Autodesk Inventor part; units mm, degrees
(part 2 of 2)
sketch "스케치7" plane through (-13.4999, 0, 82.7525) normal (-1, 0, 0) x (0, 0, -1)
  line L0 (22.7351, -5) -> (22.028, -5) projected
  line L1 (22.028, -5) -> (21.3209, -5) projected
  line L2 (21.3209, -5) -> (22.028, -5) projected
  line L3 (22.028, -5) -> (21.3209, -5) projected
  line L4 (21.3209, -5) -> (20.6138, -5) projected
  line L5 (20.6138, -5) -> (19.9067, -5) projected
  line L6 (19.9067, -5) -> (20.6138, -5) projected
  line L7 (20.6138, -5) -> (19.9067, -5) projected
  line L8 (19.9067, -5) -> (19.1996, -5) projected
  line L9 (19.1996, -5) -> (18.4924, -5) projected
  line L10 (18.4924, -5) -> (19.4924, -5) projected
  line L11 (19.4924, -5) -> (18.4924, -5) projected
  line L12 (18.4924, -5) -> (19.4924, -5) projected
  line L13 (19.4924, -5) -> (18.4924, -5) projected
  line L14 (18.4924, -5) -> (19.4924, -5) projected
  line L15 (19.4924, -5) -> (18.4924, -5) projected
  line L16 (18.4924, -5) -> (19.4924, -5) projected
  line L17 (19.4924, -5) -> (18.4924, -5) projected
  line L18 (18.4924, -5) -> (19.4924, -5) projected
  line L19 (19.4924, -5) -> (18.4924, -5) projected
  line L20 (18.4924, -5) -> (19.4924, -5) projected
  line L21 (19.4924, -5) -> (18.4924, -5) projected
  line L22 (18.4924, -5) -> (19.4924, -5) projected
  line L23 (19.4924, -5) -> (18.4924, -5) projected
  line L24 (18.4924, -5) -> (19.4924, -5) projected
  line L25 (19.4924, -5) -> (18.4924, -5) projected
  line L26 (18.4924, -5) -> (19.4924, -5) projected
  line L27 (19.4924, -5) -> (18.4924, -5) projected
  line L28 (18.4924, -5) -> (19.4924, -5) projected
  line L29 (19.4924, -5) -> (18.4924, -5) projected
  line L30 (18.4924, -5) -> (19.4924, -5) projected
  line L31 (19.4924, -5) -> (18.4924, -5) projected
  line L32 (18.4924, -5) -> (19.4924, -5) projected
  line L33 (19.4924, -5) -> (18.4924, -5) projected
  line L34 (18.4924, -5) -> (20.0726, -5) projected
  line L35 (20.0726, -5) -> (20.7798, -5) projected
  line L36 (20.7798, -5) -> (21.4869, -5) projected
  line L37 (21.4869, -5) -> (20.7798, -5) projected
  line L38 (20.7798, -5) -> (21.4869, -5) projected
  line L39 (21.4869, -5) -> (22.194, -5) projected
  line L40 (22.194, -5) -> (22.9011, -5) projected
  line L41 (22.9011, -5) -> (22.194, -5) projected
  line L42 (22.194, -5) -> (22.9011, -5) projected
  line L43 (22.9011, -5) -> (23.6082, -5) projected
  line L44 (23.6082, -5) -> (24.3153, -5) projected
  line L45 (24.3153, -5) -> (23.6082, -5) projected
  line L46 (23.6082, -5) -> (24.3153, -5) projected
  line L47 (24.3153, -5) -> (25.0224, -5) projected
  line L48 (25.0224, -5) -> (25.7295, -5) projected
  line L49 (25.7295, -5) -> (25.0224, -5) projected
  line L50 (25.0224, -5) -> (25.7295, -5) projected
  line L51 (25.7295, -5) -> (26.4366, -5) projected
  line L52 (26.4366, -5) -> (27.1437, -5) projected
  line L53 (27.1437, -5) -> (26.4366, -5) projected
  line L54 (26.4366, -5) -> (27.1437, -5) projected
  line L55 (27.1437, -5) -> (27.8508, -5) projected
  line L56 (27.8508, -5) -> (28.5579, -5) projected
  line L57 (28.5579, -5) -> (27.8508, -5) projected
  line L58 (27.8508, -5) -> (28.5579, -5) projected
  line L59 (28.5579, -5) -> (29.265, -5) projected
  line L60 (29.265, -5) -> (29.9721, -5) projected
  line L61 (29.9721, -5) -> (29.265, -5) projected
  line L62 (29.265, -5) -> (29.9721, -5) projected
  line L63 (29.9721, -5) -> (30.6792, -5) projected
  line L64 (30.6792, -5) -> (31.3864, -5) projected
  line L65 (31.3864, -5) -> (30.6792, -5) projected
  line L66 (30.6792, -5) -> (31.3864, -5) projected
  line L67 (31.3864, -5) -> (32.0935, -5) projected
  line L68 (32.0935, -5) -> (32.8006, -5) projected
  line L69 (32.8006, -5) -> (32.0935, -5) projected
  line L70 (32.0935, -5) -> (32.8006, -5) projected
  line L71 (32.8006, -5) -> (33.5077, -5) projected
  line L72 (33.5077, -5) -> (34.2148, -5) projected
  line L73 (34.2148, -5) -> (33.5077, -5) projected
  line L74 (33.5077, -5) -> (34.2148, -5) projected
  line L75 (34.2148, -5) -> (34.9219, -5) projected
  line L76 (34.9219, -5) -> (35.629, -5) projected
  line L77 (35.629, -5) -> (34.9219, -5) projected
  line L78 (34.9219, -5) -> (35.629, -5) projected
  line L79 (35.629, -5) -> (36.3361, -5) projected
  line L80 (36.3361, -5) -> (37.0432, -5) projected
  line L81 (37.0432, -5) -> (36.3361, -5) projected
  line L82 (36.3361, -5) -> (37.0432, -5) projected
  line L83 (37.0432, -5) -> (39.2779, -5) projected
  line L84 (39.2779, -5) -> (40.2779, -5) projected
  line L85 (40.2779, -5) -> (41.2779, -5) projected
  line L86 (41.2779, -5) -> (42.2779, -5) projected
  line L87 (42.2779, -5) -> (43.2779, -5) projected
  line L88 (43.2779, -5) -> (44.2779, -5) projected
  line L89 (44.2779, -5) -> (45.2779, -5) projected
  line L90 (45.2779, -5) -> (46.2779, -5) projected
  line L91 (46.2779, -5) -> (47.2779, -5) projected
  line L92 (47.2779, -5) -> (48.2779, -5) projected
  line L93 (48.2779, -5) -> (49.2779, -5) projected
  line L94 (49.2779, -5) -> (50.2779, -5) projected
  line L95 (50.2779, -5) -> (51.2779, -5) projected
  line L96 (51.2779, -5) -> (52.2779, -5) projected
  line L97 (52.2779, -5) -> (53.2779, -5) projected
  line L98 (53.2779, -5) -> (54.2779, -5) projected
  line L99 (54.2779, -5) -> (55.2779, -5) projected
  line L100 (55.2779, -5) -> (56.2779, -5) projected
  line L101 (56.2779, -5) -> (57.2779, -5) projected
  line L102 (57.2779, -5) -> (58.2779, -5) projected
  line L103 (58.2779, -5) -> (59.2779, -5) projected
  line L104 (59.2779, -5) -> (60.2779, -5) projected
  line L105 (60.2779, -5) -> (61.2779, -5) projected
  line L106 (61.2779, -5) -> (62.2779, -5) projected
  line L107 (62.2779, -5) -> (63.2779, -5) projected
  line L108 (63.2779, -5) -> (64.8581, -5) projected
  line L109 (64.8581, -5) -> (64.151, -5) projected
  line L110 (64.151, -5) -> (64.8581, -5) projected
  line L111 (64.8581, -5) -> (65.5652, -5) projected
  line L112 (65.5652, -5) -> (66.2723, -5) projected
  line L113 (66.2723, -5) -> (65.5652, -5) projected
  line L114 (65.5652, -5) -> (66.2723, -5) projected
  line L115 (66.2723, -5) -> (66.9795, -5) projected
  line L116 (66.9795, -5) -> (67.6866, -5) projected
  line L117 (67.6866, -5) -> (66.9795, -5) projected
  line L118 (66.9795, -5) -> (67.6866, -5) projected
  line L119 (67.6866, -5) -> (68.3937, -5) projected
  line L120 (68.3937, -5) -> (69.1008, -5) projected
  line L121 (69.1008, -5) -> (68.3937, -5) projected
  line L122 (68.3937, -5) -> (69.1008, -5) projected
  line L123 (69.1008, -5) -> (69.8079, -5) projected
  line L124 (69.8079, -5) -> (70.515, -5) projected
  line L125 (70.515, -5) -> (69.8079, -5) projected
  line L126 (69.8079, -5) -> (70.515, -5) projected
  line L127 (70.515, -5) -> (71.2221, -5) projected
  line L128 (71.2221, -5) -> (71.9292, -5) projected
  line L129 (71.9292, -5) -> (71.2221, -5) projected
  line L130 (71.2221, -5) -> (71.9292, -5) projected
  line L131 (71.9292, -5) -> (72.6363, -5) projected
  line L132 (72.6363, -5) -> (73.3434, -5) projected
  line L133 (73.3434, -5) -> (72.6363, -5) projected
  line L134 (72.6363, -5) -> (73.3434, -5) projected
  line L135 (73.3434, -5) -> (74.0505, -5) projected
  line L136 (74.0505, -5) -> (74.7576, -5) projected
  line L137 (74.7576, -5) -> (74.0505, -5) projected
  line L138 (74.0505, -5) -> (74.7576, -5) projected
  line L139 (74.7576, -5) -> (75.4647, -5) projected
  line L140 (75.4647, -5) -> (76.1718, -5) projected
  line L141 (76.1718, -5) -> (75.4647, -5) projected
  line L142 (75.4647, -5) -> (76.1718, -5) projected
  line L143 (76.1718, -5) -> (76.8789, -5) projected
  line L144 (76.8789, -5) -> (77.5861, -5) projected
  line L145 (77.5861, -5) -> (76.8789, -5) projected
  line L146 (76.8789, -5) -> (77.5861, -5) projected
  line L147 (77.5861, -5) -> (78.2932, -5) projected
  line L148 (78.2932, -5) -> (79.0003, -5) projected
  line L149 (79.0003, -5) -> (78.2932, -5) projected
  line L150 (78.2932, -5) -> (79.0003, -5) projected
  line L151 (79.0003, -5) -> (79.7074, -5) projected
  line L152 (79.7074, -5) -> (80.4145, -5) projected
  line L153 (80.4145, -5) -> (79.7074, -5) projected
  line L154 (79.7074, -5) -> (80.4145, -5) projected
  line L155 (80.4145, -5) -> (81.1216, -5) projected
  line L156 (81.1216, -5) -> (81.8287, -5) projected
  line L157 (81.8287, -5) -> (80.8287, -5) projected
  line L158 (80.8287, -5) -> (81.8287, -5) projected
  line L159 (81.8287, -5) -> (80.8287, -5) projected
  line L160 (80.8287, -5) -> (81.8287, -5) projected
  line L161 (81.8287, -5) -> (80.8287, -5) projected
  line L162 (80.8287, -5) -> (81.8287, -5) projected
  line L163 (81.8287, -5) -> (80.8287, -5) projected
  line L164 (80.8287, -5) -> (81.8287, -5) projected
  line L165 (81.8287, -5) -> (80.8287, -5) projected
  line L166 (80.8287, -5) -> (81.8287, -5) projected
  line L167 (81.8287, -5) -> (80.8287, -5) projected
  line L168 (80.8287, -5) -> (81.8287, -5) projected
  line L169 (81.8287, -5) -> (80.8287, -5) projected
  line L170 (80.8287, -5) -> (81.8287, -5) projected
  line L171 (81.8287, -5) -> (80.8287, -5) projected
  line L172 (80.8287, -5) -> (81.8287, -5) projected
  line L173 (81.8287, -5) -> (80.8287, -5) projected
  line L174 (80.8287, -5) -> (81.8287, -5) projected
  line L175 (81.8287, -5) -> (80.8287, -5) projected
  line L176 (80.8287, -5) -> (81.8287, -5) projected
  line L177 (81.8287, -5) -> (80.8287, -5) projected
  line L178 (80.8287, -5) -> (81.8287, -5) projected
  line L179 (81.8287, -5) -> (80.8287, -5) projected
  line L180 (80.8287, -5) -> (81.8287, -5) projected
  line L181 (81.8287, -5) -> (80.2485, -5) projected
  line L182 (80.2485, -5) -> (79.5414, -5) projected
  line L183 (79.5414, -5) -> (78.8343, -5) projected
  line L184 (78.8343, -5) -> (79.5414, -5) projected
  line L185 (79.5414, -5) -> (78.8343, -5) projected
  line L186 (78.8343, -5) -> (78.1272, -5) projected
  line L187 (78.1272, -5) -> (77.4201, -5) projected
  line L188 (77.4201, -5) -> (78.1272, -5) projected
  line L189 (78.1272, -5) -> (77.4201, -5) projected
  line L190 (77.4201, -5) -> (76.713, -5) projected
  line L191 (76.713, -5) -> (76.0059, -5) projected
  line L192 (76.0059, -5) -> (76.713, -5) projected
  line L193 (76.713, -5) -> (76.0059, -5) projected
  line L194 (76.0059, -5) -> (75.2988, -5) projected
  line L195 (75.2988, -5) -> (74.5916, -5) projected
  line L196 (74.5916, -5) -> (75.2988, -5) projected
  line L197 (75.2988, -5) -> (74.5916, -5) projected
  line L198 (74.5916, -5) -> (73.8845, -5) projected
  line L199 (73.8845, -5) -> (73.1774, -5) projected
  line L200 (73.1774, -5) -> (73.8845, -5) projected
  line L201 (73.8845, -5) -> (73.1774, -5) projected
  line L202 (73.1774, -5) -> (72.4703, -5) projected
  line L203 (72.4703, -5) -> (71.7632, -5) projected
  line L204 (71.7632, -5) -> (72.4703, -5) projected
  line L205 (72.4703, -5) -> (71.7632, -5) projected
  line L206 (71.7632, -5) -> (71.0561, -5) projected
  line L207 (71.0561, -5) -> (70.349, -5) projected
  line L208 (70.349, -5) -> (71.0561, -5) projected
  line L209 (71.0561, -5) -> (70.349, -5) projected
  line L210 (70.349, -5) -> (69.6419, -5) projected
  line L211 (69.6419, -5) -> (68.9348, -5) projected
  line L212 (68.9348, -5) -> (69.6419, -5) projected
  line L213 (69.6419, -5) -> (68.9348, -5) projected
  line L214 (68.9348, -5) -> (68.2277, -5) projected
  line L215 (68.2277, -5) -> (67.5206, -5) projected
  line L216 (67.5206, -5) -> (68.2277, -5) projected
  line L217 (68.2277, -5) -> (67.5206, -5) projected
  line L218 (67.5206, -5) -> (66.8135, -5) projected
  line L219 (66.8135, -5) -> (66.1064, -5) projected
  line L220 (66.1064, -5) -> (66.8135, -5) projected
  line L221 (66.8135, -5) -> (66.1064, -5) projected
  line L222 (66.1064, -5) -> (65.3993, -5) projected
  line L223 (65.3993, -5) -> (64.6922, -5) projected
  line L224 (64.6922, -5) -> (65.3993, -5) projected
  line L225 (65.3993, -5) -> (64.6922, -5) projected
  line L226 (64.6922, -5) -> (63.985, -5) projected
  line L227 (63.985, -5) -> (63.2779, -5) projected
  line L228 (63.2779, -5) -> (63.985, -5) projected
  line L229 (63.985, -5) -> (63.2779, -5) projected
  line L230 (63.2779, -5) -> (61.0432, -5) projected
  line L231 (61.0432, -5) -> (60.0432, -5) projected
  line L232 (60.0432, -5) -> (59.0432, -5) projected
  line L233 (59.0432, -5) -> (58.0432, -5) projected
  line L234 (58.0432, -5) -> (57.0432, -5) projected
  line L235 (57.0432, -5) -> (56.0432, -5) projected
  line L236 (56.0432, -5) -> (55.0432, -5) projected
  line L237 (55.0432, -5) -> (54.0432, -5) projected
  line L238 (54.0432, -5) -> (53.0432, -5) projected
  line L239 (53.0432, -5) -> (52.0432, -5) projected
  line L240 (52.0432, -5) -> (51.0432, -5) projected
  line L241 (51.0432, -5) -> (50.0432, -5) projected
  line L242 (50.0432, -5) -> (49.0432, -5) projected
  line L243 (49.0432, -5) -> (48.0432, -5) projected
  line L244 (48.0432, -5) -> (47.0432, -5) projected
  line L245 (47.0432, -5) -> (46.0432, -5) projected
  line L246 (46.0432, -5) -> (45.0432, -5) projected
  line L247 (45.0432, -5) -> (44.0432, -5) projected
  line L248 (44.0432, -5) -> (43.0432, -5) projected
  line L249 (43.0432, -5) -> (42.0432, -5) projected
  line L250 (42.0432, -5) -> (41.0432, -5) projected
  line L251 (41.0432, -5) -> (40.0432, -5) projected
  line L252 (40.0432, -5) -> (39.0432, -5) projected
  line L253 (39.0432, -5) -> (38.0432, -5) projected
  line L254 (38.0432, -5) -> (37.0432, -5) projected
  line L255 (37.0432, -5) -> (35.463, -5) projected
  line L256 (35.463, -5) -> (36.1701, -5) projected
  line L257 (36.1701, -5) -> (35.463, -5) projected
  line L258 (35.463, -5) -> (34.7559, -5) projected
  line L259 (34.7559, -5) -> (34.0488, -5) projected
  line L260 (34.0488, -5) -> (34.7559, -5) projected
  line L261 (34.7559, -5) -> (34.0488, -5) projected
  line L262 (34.0488, -5) -> (33.3417, -5) projected
  line L263 (33.3417, -5) -> (32.6346, -5) projected
  line L264 (32.6346, -5) -> (33.3417, -5) projected
  line L265 (33.3417, -5) -> (32.6346, -5) projected
  line L266 (32.6346, -5) -> (31.9275, -5) projected
  line L267 (31.9275, -5) -> (31.2204, -5) projected
  line L268 (31.2204, -5) -> (31.9275, -5) projected
  line L269 (31.9275, -5) -> (31.2204, -5) projected
  line L270 (31.2204, -5) -> (30.5133, -5) projected
  line L271 (30.5133, -5) -> (29.8062, -5) projected
  line L272 (29.8062, -5) -> (30.5133, -5) projected
  line L273 (30.5133, -5) -> (29.8062, -5) projected
  line L274 (29.8062, -5) -> (29.0991, -5) projected
  line L275 (29.0991, -5) -> (28.3919, -5) projected
  line L276 (28.3919, -5) -> (29.0991, -5) projected
  line L277 (29.0991, -5) -> (28.3919, -5) projected
  line L278 (28.3919, -5) -> (27.6848, -5) projected
  line L279 (27.6848, -5) -> (26.9777, -5) projected
  line L280 (26.9777, -5) -> (27.6848, -5) projected
  line L281 (27.6848, -5) -> (26.9777, -5) projected
  line L282 (26.9777, -5) -> (26.2706, -5) projected
  line L283 (26.2706, -5) -> (25.5635, -5) projected
  line L284 (25.5635, -5) -> (26.2706, -5) projected
  line L285 (26.2706, -5) -> (25.5635, -5) projected
  line L286 (25.5635, -5) -> (24.8564, -5) projected
  line L287 (24.8564, -5) -> (24.1493, -5) projected
  line L288 (24.1493, -5) -> (24.8564, -5) projected
  line L289 (24.8564, -5) -> (24.1493, -5) projected
  line L290 (24.1493, -5) -> (23.4422, -5) projected
  line L291 (23.4422, -5) -> (22.7351, -5) projected
  line L292 (22.7351, -5) -> (23.4422, -5) projected
  line L293 (23.4422, -5) -> (22.7351, -5) projected
  line L294 (22.7351, 0) -> (22.028, 0) projected
  line L295 (23.4422, 0) -> (22.7351, 0) projected
  line L296 (22.7351, 0) -> (23.4422, 0) projected
  line L297 (23.4422, 0) -> (22.7351, 0) projected
  line L298 (24.1493, 0) -> (23.4422, 0) projected
  line L299 (24.8564, 0) -> (24.1493, 0) projected
  line L300 (24.1493, 0) -> (24.8564, 0) projected
  line L301 (24.8564, 0) -> (24.1493, 0) projected
  line L302 (25.5635, 0) -> (24.8564, 0) projected
  line L303 (26.2706, 0) -> (25.5635, 0) projected
  line L304 (25.5635, 0) -> (26.2706, 0) projected
  line L305 (26.2706, 0) -> (25.5635, 0) projected
  line L306 (26.9777, 0) -> (26.2706, 0) projected
  line L307 (27.6848, 0) -> (26.9777, 0) projected
  line L308 (26.9777, 0) -> (27.6848, 0) projected
  line L309 (27.6848, 0) -> (26.9777, 0) projected
  line L310 (28.3919, 0) -> (27.6848, 0) projected
  line L311 (29.0991, 0) -> (28.3919, 0) projected
  line L312 (28.3919, 0) -> (29.0991, 0) projected
  line L313 (29.0991, 0) -> (28.3919, 0) projected
  line L314 (29.8062, 0) -> (29.0991, 0) projected
  line L315 (30.5133, 0) -> (29.8062, 0) projected
  line L316 (29.8062, 0) -> (30.5133, 0) projected
  line L317 (30.5133, 0) -> (29.8062, 0) projected
  line L318 (31.2204, 0) -> (30.5133, 0) projected
  line L319 (31.9275, 0) -> (31.2204, 0) projected
  line L320 (31.2204, 0) -> (31.9275, 0) projected
  line L321 (31.9275, 0) -> (31.2204, 0) projected
  line L322 (32.6346, 0) -> (31.9275, 0) projected
  line L323 (33.3417, 0) -> (32.6346, 0) projected
  line L324 (32.6346, 0) -> (33.3417, 0) projected
  line L325 (33.3417, 0) -> (32.6346, 0) projected
  line L326 (34.0488, 0) -> (33.3417, 0) projected
  line L327 (34.7559, 0) -> (34.0488, 0) projected
  line L328 (34.0488, 0) -> (34.7559, 0) projected
  line L329 (34.7559, 0) -> (34.0488, 0) projected
  line L330 (35.463, 0) -> (34.7559, 0) projected
  line L331 (36.1701, 0) -> (35.463, 0) projected
  line L332 (35.463, 0) -> (36.1701, 0) projected
  line L333 (37.0432, 0) -> (35.463, 0) projected
  line L334 (38.0432, 0) -> (37.0432, 0) projected
  line L335 (39.0432, 0) -> (38.0432, 0) projected
  line L336 (40.0432, 0) -> (39.0432, 0) projected
  line L337 (41.0432, 0) -> (40.0432, 0) projected
  line L338 (42.0432, 0) -> (41.0432, 0) projected
  line L339 (43.0432, 0) -> (42.0432, 0) projected
  line L340 (44.0432, 0) -> (43.0432, 0) projected
  line L341 (45.0432, 0) -> (44.0432, 0) projected
  line L342 (46.0432, 0) -> (45.0432, 0) projected
  line L343 (47.0432, 0) -> (46.0432, 0) projected
  line L344 (48.0432, 0) -> (47.0432, 0) projected
  line L345 (49.0432, 0) -> (48.0432, 0) projected
  line L346 (50.0432, 0) -> (49.0432, 0) projected
  line L347 (51.0432, 0) -> (50.0432, 0) projected
  line L348 (52.0432, 0) -> (51.0432, 0) projected
  line L349 (53.0432, 0) -> (52.0432, 0) projected
  line L350 (54.0432, 0) -> (53.0432, 0) projected
  line L351 (55.0432, 0) -> (54.0432, 0) projected
  line L352 (56.0432, 0) -> (55.0432, 0) projected
  line L353 (57.0432, 0) -> (56.0432, 0) projected
  line L354 (58.0432, 0) -> (57.0432, 0) projected
  line L355 (59.0432, 0) -> (58.0432, 0) projected
  line L356 (60.0432, 0) -> (59.0432, 0) projected
  line L357 (61.0432, 0) -> (60.0432, 0) projected
  line L358 (63.2779, 0) -> (61.0432, 0) projected
  line L359 (63.985, 0) -> (63.2779, 0) projected
  line L360 (63.2779, 0) -> (63.985, 0) projected
  line L361 (63.985, 0) -> (63.2779, 0) projected
  line L362 (64.6922, 0) -> (63.985, 0) projected
  line L363 (65.3993, 0) -> (64.6922, 0) projected
  line L364 (64.6922, 0) -> (65.3993, 0) projected
  line L365 (65.3993, 0) -> (64.6922, 0) projected
  line L366 (66.1064, 0) -> (65.3993, 0) projected
  line L367 (66.8135, 0) -> (66.1064, 0) projected
  line L368 (66.1064, 0) -> (66.8135, 0) projected
  line L369 (66.8135, 0) -> (66.1064, 0) projected
  line L370 (67.5206, 0) -> (66.8135, 0) projected
  line L371 (68.2277, 0) -> (67.5206, 0) projected
  line L372 (67.5206, 0) -> (68.2277, 0) projected
  line L373 (68.2277, 0) -> (67.5206, 0) projected
  line L374 (68.9348, 0) -> (68.2277, 0) projected
  line L375 (69.6419, 0) -> (68.9348, 0) projected
  line L376 (68.9348, 0) -> (69.6419, 0) projected
  line L377 (69.6419, 0) -> (68.9348, 0) projected
  line L378 (70.349, 0) -> (69.6419, 0) projected
  line L379 (71.0561, 0) -> (70.349, 0) projected
  line L380 (70.349, 0) -> (71.0561, 0) projected
  line L381 (71.0561, 0) -> (70.349, 0) projected
  line L382 (71.7632, 0) -> (71.0561, 0) projected
  line L383 (72.4703, 0) -> (71.7632, 0) projected
  line L384 (71.7632, 0) -> (72.4703, 0) projected
  line L385 (72.4703, 0) -> (71.7632, 0) projected
  line L386 (73.1774, 0) -> (72.4703, 0) projected
  line L387 (73.8845, 0) -> (73.1774, 0) projected
  line L388 (73.1774, 0) -> (73.8845, 0) projected
  line L389 (73.8845, 0) -> (73.1774, 0) projected
  line L390 (74.5916, 0) -> (73.8845, 0) projected
  line L391 (75.2988, 0) -> (74.5916, 0) projected
  line L392 (74.5916, 0) -> (75.2988, 0) projected
  line L393 (75.2988, 0) -> (74.5916, 0) projected
  line L394 (76.0059, 0) -> (75.2988, 0) projected
  line L395 (76.713, 0) -> (76.0059, 0) projected
  line L396 (76.0059, 0) -> (76.713, 0) projected
  line L397 (76.713, 0) -> (76.0059, 0) projected
  line L398 (77.4201, 0) -> (76.713, 0) projected
  line L399 (78.1272, 0) -> (77.4201, 0) projected
  line L400 (77.4201, 0) -> (78.1272, 0) projected
  line L401 (78.1272, 0) -> (77.4201, 0) projected
  line L402 (78.8343, 0) -> (78.1272, 0) projected
  line L403 (79.5414, 0) -> (78.8343, 0) projected
  line L404 (78.8343, 0) -> (79.5414, 0) projected
  line L405 (79.5414, 0) -> (78.8343, 0) projected
  line L406 (80.2485, 0) -> (79.5414, 0) projected
  line L407 (81.8287, 0) -> (80.2485, 0) projected
  line L408 (80.8287, 0) -> (81.8287, 0) projected
  line L409 (81.8287, 0) -> (80.8287, 0) projected
  line L410 (80.8287, 0) -> (81.8287, 0) projected
  line L411 (81.8287, 0) -> (80.8287, 0) projected
  line L412 (80.8287, 0) -> (81.8287, 0) projected
  line L413 (81.8287, 0) -> (80.8287, 0) projected
  line L414 (80.8287, 0) -> (81.8287, 0) projected
  line L415 (81.8287, 0) -> (80.8287, 0) projected
  line L416 (80.8287, 0) -> (81.8287, 0) projected
  line L417 (81.8287, 0) -> (80.8287, 0) projected
  line L418 (80.8287, 0) -> (81.8287, 0) projected
  line L419 (81.8287, 0) -> (80.8287, 0) projected
  line L420 (80.8287, 0) -> (81.8287, 0) projected
  line L421 (81.8287, 0) -> (80.8287, 0) projected
  line L422 (80.8287, 0) -> (81.8287, 0) projected
  line L423 (81.8287, 0) -> (80.8287, 0) projected
  line L424 (80.8287, 0) -> (81.8287, 0) projected
  line L425 (81.8287, 0) -> (80.8287, 0) projected
  line L426 (80.8287, 0) -> (81.8287, 0) projected
  line L427 (81.8287, 0) -> (80.8287, 0) projected
  line L428 (80.8287, 0) -> (81.8287, 0) projected
  line L429 (81.8287, 0) -> (80.8287, 0) projected
  line L430 (80.8287, 0) -> (81.8287, 0) projected
  line L431 (81.8287, 0) -> (80.8287, 0) projected
  line L432 (81.1216, 0) -> (81.8287, 0) projected
  line L433 (80.4145, 0) -> (81.1216, 0) projected
  line L434 (79.7074, 0) -> (80.4145, 0) projected
  line L435 (80.4145, 0) -> (79.7074, 0) projected
  line L436 (79.7074, 0) -> (80.4145, 0) projected
  line L437 (79.0003, 0) -> (79.7074, 0) projected
  line L438 (78.2932, 0) -> (79.0003, 0) projected
  line L439 (79.0003, 0) -> (78.2932, 0) projected
  line L440 (78.2932, 0) -> (79.0003, 0) projected
  line L441 (77.5861, 0) -> (78.2932, 0) projected
  line L442 (76.8789, 0) -> (77.5861, 0) projected
  line L443 (77.5861, 0) -> (76.8789, 0) projected
  line L444 (76.8789, 0) -> (77.5861, 0) projected
  line L445 (76.1718, 0) -> (76.8789, 0) projected
  line L446 (75.4647, 0) -> (76.1718, 0) projected
  line L447 (76.1718, 0) -> (75.4647, 0) projected
  line L448 (75.4647, 0) -> (76.1718, 0) projected
  line L449 (74.7576, 0) -> (75.4647, 0) projected
  line L450 (74.0505, 0) -> (74.7576, 0) projected
  line L451 (74.7576, 0) -> (74.0505, 0) projected
  line L452 (74.0505, 0) -> (74.7576, 0) projected
  line L453 (73.3434, 0) -> (74.0505, 0) projected
  line L454 (72.6363, 0) -> (73.3434, 0) projected
  line L455 (73.3434, 0) -> (72.6363, 0) projected
  line L456 (72.6363, 0) -> (73.3434, 0) projected
  line L457 (71.9292, 0) -> (72.6363, 0) projected
  line L458 (71.2221, 0) -> (71.9292, 0) projected
  line L459 (71.9292, 0) -> (71.2221, 0) projected
  line L460 (71.2221, 0) -> (71.9292, 0) projected
  line L461 (70.515, 0) -> (71.2221, 0) projected
  line L462 (69.8079, 0) -> (70.515, 0) projected
  line L463 (70.515, 0) -> (69.8079, 0) projected
  line L464 (69.8079, 0) -> (70.515, 0) projected
  line L465 (69.1008, 0) -> (69.8079, 0) projected
  line L466 (68.3937, 0) -> (69.1008, 0) projected
  line L467 (69.1008, 0) -> (68.3937, 0) projected
  line L468 (68.3937, 0) -> (69.1008, 0) projected
  line L469 (67.6866, 0) -> (68.3937, 0) projected
  line L470 (66.9795, 0) -> (67.6866, 0) projected
  line L471 (67.6866, 0) -> (66.9795, 0) projected
  line L472 (66.9795, 0) -> (67.6866, 0) projected
  line L473 (66.2723, 0) -> (66.9795, 0) projected
  line L474 (65.5652, 0) -> (66.2723, 0) projected
  line L475 (66.2723, 0) -> (65.5652, 0) projected
  line L476 (65.5652, 0) -> (66.2723, 0) projected
  line L477 (64.8581, 0) -> (65.5652, 0) projected
  line L478 (64.151, 0) -> (64.8581, 0) projected
  line L479 (64.8581, 0) -> (64.151, 0) projected
  line L480 (63.2779, 0) -> (64.8581, 0) projected
  line L481 (62.2779, 0) -> (63.2779, 0) projected
  line L482 (61.2779, 0) -> (62.2779, 0) projected
  line L483 (60.2779, 0) -> (61.2779, 0) projected
  line L484 (59.2779, 0) -> (60.2779, 0) projected
  line L485 (58.2779, 0) -> (59.2779, 0) projected
  line L486 (57.2779, 0) -> (58.2779, 0) projected
  line L487 (56.2779, 0) -> (57.2779, 0) projected
  line L488 (55.2779, 0) -> (56.2779, 0) projected
  line L489 (54.2779, 0) -> (55.2779, 0) projected
  line L490 (53.2779, 0) -> (54.2779, 0) projected
  line L491 (52.2779, 0) -> (53.2779, 0) projected
  line L492 (51.2779, 0) -> (52.2779, 0) projected
  line L493 (50.2779, 0) -> (51.2779, 0) projected
  line L494 (49.2779, 0) -> (50.2779, 0) projected
  line L495 (48.2779, 0) -> (49.2779, 0) projected
  line L496 (47.2779, 0) -> (48.2779, 0) projected
  line L497 (46.2779, 0) -> (47.2779, 0) projected
  line L498 (45.2779, 0) -> (46.2779, 0) projected
  line L499 (44.2779, 0) -> (45.2779, 0) projected
  line L500 (43.2779, 0) -> (44.2779, 0) projected
  line L501 (42.2779, 0) -> (43.2779, 0) projected
  line L502 (41.2779, 0) -> (42.2779, 0) projected
  line L503 (40.2779, 0) -> (41.2779, 0) projected
  line L504 (39.2779, 0) -> (40.2779, 0) projected
  line L505 (37.0432, 0) -> (39.2779, 0) projected
  line L506 (36.3361, 0) -> (37.0432, 0) projected
  line L507 (37.0432, 0) -> (36.3361, 0) projected
  line L508 (36.3361, 0) -> (37.0432, 0) projected
  line L509 (35.629, 0) -> (36.3361, 0) projected
  line L510 (34.9219, 0) -> (35.629, 0) projected
  line L511 (35.629, 0) -> (34.9219, 0) projected
  line L512 (34.9219, 0) -> (35.629, 0) projected
  line L513 (34.2148, 0) -> (34.9219, 0) projected
  line L514 (33.5077, 0) -> (34.2148, 0) projected
  line L515 (34.2148, 0) -> (33.5077, 0) projected
  line L516 (33.5077, 0) -> (34.2148, 0) projected
  line L517 (32.8006, 0) -> (33.5077, 0) projected
  line L518 (32.0935, 0) -> (32.8006, 0) projected
  line L519 (32.8006, 0) -> (32.0935, 0) projected
  line L520 (32.0935, 0) -> (32.8006, 0) projected
  line L521 (31.3864, 0) -> (32.0935, 0) projected
  line L522 (30.6792, 0) -> (31.3864, 0) projected
  line L523 (31.3864, 0) -> (30.6792, 0) projected
  line L524 (30.6792, 0) -> (31.3864, 0) projected
  line L525 (29.9721, 0) -> (30.6792, 0) projected
  line L526 (29.265, 0) -> (29.9721, 0) projected
  line L527 (29.9721, 0) -> (29.265, 0) projected
  line L528 (29.265, 0) -> (29.9721, 0) projected
  line L529 (28.5579, 0) -> (29.265, 0) projected
  line L530 (27.8508, 0) -> (28.5579, 0) projected
  line L531 (28.5579, 0) -> (27.8508, 0) projected
  line L532 (27.8508, 0) -> (28.5579, 0) projected
  line L533 (27.1437, 0) -> (27.8508, 0) projected
  line L534 (26.4366, 0) -> (27.1437, 0) projected
  line L535 (27.1437, 0) -> (26.4366, 0) projected
  line L536 (26.4366, 0) -> (27.1437, 0) projected
  line L537 (25.7295, 0) -> (26.4366, 0) projected
  line L538 (25.0224, 0) -> (25.7295, 0) projected
  line L539 (25.7295, 0) -> (25.0224, 0) projected
  line L540 (25.0224, 0) -> (25.7295, 0) projected
  line L541 (24.3153, 0) -> (25.0224, 0) projected
  line L542 (23.6082, 0) -> (24.3153, 0) projected
  line L543 (24.3153, 0) -> (23.6082, 0) projected
  line L544 (23.6082, 0) -> (24.3153, 0) projected
  line L545 (22.9011, 0) -> (23.6082, 0) projected
  line L546 (22.194, 0) -> (22.9011, 0) projected
  line L547 (22.9011, 0) -> (22.194, 0) projected
  line L548 (22.194, 0) -> (22.9011, 0) projected
  line L549 (21.4869, 0) -> (22.194, 0) projected
  line L550 (20.7798, 0) -> (21.4869, 0) projected
  line L551 (21.4869, 0) -> (20.7798, 0) projected
  line L552 (20.7798, 0) -> (21.4869, 0) projected
  line L553 (20.0726, 0) -> (20.7798, 0) projected
  line L554 (18.4924, 0) -> (20.0726, 0) projected
  line L555 (19.4924, 0) -> (18.4924, 0) projected
  line L556 (18.4924, 0) -> (19.4924, 0) projected
  line L557 (19.4924, 0) -> (18.4924, 0) projected
  line L558 (18.4924, 0) -> (19.4924, 0) projected
  line L559 (19.4924, 0) -> (18.4924, 0) projected
  line L560 (18.4924, 0) -> (19.4924, 0) projected
  line L561 (19.4924, 0) -> (18.4924, 0) projected
  line L562 (18.4924, 0) -> (19.4924, 0) projected
  line L563 (19.4924, 0) -> (18.4924, 0) projected
  line L564 (18.4924, 0) -> (19.4924, 0) projected
  line L565 (19.4924, 0) -> (18.4924, 0) projected
  line L566 (18.4924, 0) -> (19.4924, 0) projected
  line L567 (19.4924, 0) -> (18.4924, 0) projected
  line L568 (18.4924, 0) -> (19.4924, 0) projected
  line L569 (19.4924, 0) -> (18.4924, 0) projected
  line L570 (18.4924, 0) -> (19.4924, 0) projected
  line L571 (19.4924, 0) -> (18.4924, 0) projected
  line L572 (18.4924, 0) -> (19.4924, 0) projected
  line L573 (19.4924, 0) -> (18.4924, 0) projected
  line L574 (18.4924, 0) -> (19.4924, 0) projected
  line L575 (19.4924, 0) -> (18.4924, 0) projected
  line L576 (18.4924, 0) -> (19.4924, 0) projected
  line L577 (19.4924, 0) -> (18.4924, 0) projected
  line L578 (18.4924, 0) -> (19.4924, 0) projected
  line L579 (19.1996, 0) -> (18.4924, 0) projected
  line L580 (19.9067, 0) -> (19.1996, 0) projected
  line L581 (20.6138, 0) -> (19.9067, 0) projected
  line L582 (19.9067, 0) -> (20.6138, 0) projected
  line L583 (20.6138, 0) -> (19.9067, 0) projected
  line L584 (21.3209, 0) -> (20.6138, 0) projected
  line L585 (22.028, 0) -> (21.3209, 0) projected
  line L586 (21.3209, 0) -> (22.028, 0) projected
  line L587 (22.028, 0) -> (21.3209, 0) projected
  line L588 (40.1604, 10) -> (60.1604, 10)
  line L589 (60.1604, 10) -> (60.1604, 0)
  line L590 (60.1604, 0) -> (40.1604, 0)
  line L591 (40.1604, 0) -> (40.1604, 10)
  circle A0 centre (45.1604, 5) radius 1.25
  circle A1 centre (55.1604, 5) radius 1.25
  point P0 (82.7525, 0)
  point P1 (50.1604, 0)
  point P2 (50.1604, 0)
  point P3 (50.1604, 0)
  point P4 (50.1604, 10)
  point P5 (48.0432, 0)
  point P6 (49.0432, 0)
  point P7 (50.0432, 0)
  point P8 (51.0432, 0)
  point P9 (52.0432, 0)
  point P10 (53.0432, 0)
  point P11 (54.0432, 0)
  point P12 (55.0432, 0)
  point P13 (56.0432, 0)
  point P14 (57.0432, 0)
  point P15 (58.0432, 0)
  point P16 (59.0432, 0)
  point P17 (60.0432, 0)
  dimension "d18" = 20
  dimension "d19" = 10
  dimension "d20" = 0
  dimension "d21" = 2.5
  dimension "d22" = 2.5
  dimension "d23" = 5
  dimension "d24" = 5
  dimension "d25" = 5
  dimension "d26" = 5
  constraints: 8 end point, 2 centre point, 2 parallel, 1 horizontal, 1 midpoint, 1 perpendicular, 1 vertical alignment
  measures "d18" distance of L589.end L590.end
  measures "d19" distance of L588.end L589.end
  measures "d20" distance from line of L351.start L590
  measures "d21" diameter of A0
  measures "d22" diameter of A1
  measures "d23" distance from line of L588 A0.centre
  measures "d24" distance from line of L591 A0.centre
  measures "d25" distance from line of L588 A1.centre
  measures "d26" distance from line of L589 A1.centre
extrude "돌출3" add sketch "스케치7" along normal mid plane 15
sketch "스케치8" plane through (-20.9999, -10, 42.592) normal (0, -1, 0) x (1, 0, 0)
  line L0 (0, 0) -> (15, 0) projected
  line L1 (0, -20) -> (0, 0) projected
  line L2 (15, -20) -> (0, -20) projected
  line L3 (15, 0) -> (15, -20) projected
  line L4 (0, 0) -> (15, 0) projected
  line L5 (5, 0) -> (5, -20)
  line L6 (15, -20) -> (0, -20) projected
  line L7 (10, -20) -> (10, 0)
  point P0 (20.9999, -42.592)
  dimension "d29" = 5
  dimension "d30" = 5
  constraints: 4 end point, 4 point on line, 2 perpendicular
  measures "d29" distance between parallel lines of L3 L7
  measures "d30" distance between parallel lines of L1 L5
extrude "돌출4" cut sketch "스케치8" against normal up to surface (10 mm away) contours L0 L7 L2 L5
